Autodesk Fusion 360 part; units mm, degrees
(part 2 of 2)
sketch "lateral-dxf-sketch" plane through (0, 0, 0) normal (0, 1, 0) x (1, 0, 0) in component "Lateral Panel"
  line L0 (153.5, 5) -> (153.5, -5)
  line L1 (153.5, -5) -> (157, -5)
  line L2 (157, -5) -> (157, -15)
  line L3 (157, -15) -> (153.5, -15)
  line L4 (153.5, -15) -> (153.5, -30)
  line L5 (153.5, -30) -> (53.5, -30)
  line L6 (53.5, -30) -> (53.5, 15)
  line L7 (53.5, 15) -> (50, 15)
  line L8 (50, 15) -> (50, -30)
  line L9 (50, -30) -> (-50, -30)
  line L10 (-50, -30) -> (-50, 15)
  line L11 (-50, 15) -> (-53.5, 15)
  line L12 (-53.5, 15) -> (-53.5, -30)
  line L13 (-53.5, -30) -> (-153.5, -30)
  line L14 (-153.5, -30) -> (-153.5, -15)
  line L15 (-153.5, -15) -> (-157, -15)
  line L16 (-157, -15) -> (-157, -5)
  line L17 (-157, -5) -> (-153.5, -5)
  line L18 (-153.5, -5) -> (-153.5, 5)
  line L19 (-153.5, 5) -> (-157, 5)
  line L20 (-157, 5) -> (-157, 15)
  line L21 (-157, 15) -> (-153.5, 15)
  line L22 (-153.5, 15) -> (-153.5, 30)
  line L23 (-153.5, 30) -> (153.5, 30)
  line L24 (153.5, 30) -> (153.5, 15)
  line L25 (153.5, 15) -> (157, 15)
  line L26 (157, 15) -> (157, 5)
  line L27 (157, 5) -> (153.5, 5)
extrude "Extrude1'" add sketch "Sketch1" along normal blind 3.5 separate body makes body 3 in component "Side Panel"
sketch "side-panel-dxf-sketch" plane through (0, 0, 0) normal (0, 1, 0) x (1, 0, 0) in component "Side Panel"
  line L0 (72.2516, -98.9992) -> (68.7516, -98.9992)
  line L1 (68.7516, -98.9992) -> (68.7516, -108.9992)
  line L2 (68.7516, -108.9992) -> (72.2516, -108.9992)
  line L3 (72.2516, -108.9992) -> (72.2516, -98.9992)
  line L4 (213.25, -57) -> (213.25, -47)
  line L5 (213.25, -47) -> (209.75, -47)
  line L6 (209.75, -47) -> (209.75, -57)
  line L7 (209.75, -57) -> (213.25, -57)
  line L8 (213.25, -37) -> (213.25, -27)
  line L9 (213.25, -27) -> (209.75, -27)
  line L10 (209.75, -27) -> (209.75, -37)
  line L11 (209.75, -37) -> (213.25, -37)
  line L12 (189.7503, -38.9999) -> (186.2503, -38.9999)
  line L13 (186.2503, -38.9999) -> (186.2503, -48.9999)
  line L14 (186.2503, -48.9999) -> (189.7503, -48.9999)
  line L15 (189.7503, -48.9999) -> (189.7503, -38.9999)
  line L16 (186.2503, -58.9999) -> (186.2503, -68.9999)
  line L17 (186.2503, -68.9999) -> (189.7503, -68.9999)
  line L18 (189.7503, -68.9999) -> (189.7503, -58.9999)
  line L19 (189.7503, -58.9999) -> (186.2503, -58.9999)
  line L20 (166.2505, -50.9997) -> (162.7505, -50.9997)
  line L21 (162.7505, -50.9997) -> (162.7505, -60.9997)
  line L22 (162.7505, -60.9997) -> (166.2505, -60.9997)
  line L23 (166.2505, -60.9997) -> (166.2505, -50.9997)
  line L24 (162.7505, -70.9997) -> (162.7505, -80.9997)
  line L25 (162.7505, -80.9997) -> (166.2505, -80.9997)
  line L26 (166.2505, -80.9997) -> (166.2505, -70.9997)
  line L27 (166.2505, -70.9997) -> (162.7505, -70.9997)
  line L28 (142.7508, -62.9996) -> (139.2508, -62.9996)
  line L29 (139.2508, -62.9996) -> (139.2508, -72.9996)
  line L30 (139.2508, -72.9996) -> (142.7508, -72.9996)
  line L31 (142.7508, -72.9996) -> (142.7508, -62.9996)
  line L32 (139.2508, -82.9996) -> (139.2508, -92.9996)
  line L33 (139.2508, -92.9996) -> (142.7508, -92.9996)
  line L34 (142.7508, -92.9996) -> (142.7508, -82.9996)
  line L35 (142.7508, -82.9996) -> (139.2508, -82.9996)
  line L36 (119.2511, -74.9995) -> (115.7511, -74.9995)
  line L37 (115.7511, -74.9995) -> (115.7511, -84.9995)
  line L38 (115.7511, -84.9995) -> (119.2511, -84.9995)
  line L39 (119.2511, -84.9995) -> (119.2511, -74.9995)
  line L40 (92.2513, -106.9993) -> (92.2513, -116.9993)
  line L41 (92.2513, -116.9993) -> (95.7513, -116.9993)
  line L42 (95.7513, -116.9993) -> (95.7513, -106.9993)
  line L43 (95.7513, -106.9993) -> (92.2513, -106.9993)
  line L44 (-1.75, -15) -> (-1.75, -25)
  line L45 (-1.75, -25) -> (1.75, -25)
  line L46 (1.75, -25) -> (1.75, -15)
  line L47 (1.75, -15) -> (-1.75, -15)
  line L48 (-1.75, -55) -> (-1.75, -65)
  line L49 (-1.75, -65) -> (1.75, -65)
  line L50 (1.75, -65) -> (1.75, -55)
  line L51 (1.75, -55) -> (-1.75, -55)
  line L52 (95.7513, -86.9993) -> (92.2513, -86.9993)
  line L53 (92.2513, -86.9993) -> (92.2513, -96.9993)
  line L54 (92.2513, -96.9993) -> (95.7513, -96.9993)
  line L55 (95.7513, -96.9993) -> (95.7513, -86.9993)
  line L56 (115.7511, -94.9995) -> (115.7511, -104.9995)
  line L57 (115.7511, -104.9995) -> (119.2511, -104.9995)
  line L58 (119.2511, -104.9995) -> (119.2511, -94.9995)
  line L59 (119.2511, -94.9995) -> (115.7511, -94.9995)
  line L60 (68.7516, -118.9992) -> (68.7516, -128.9992)
  line L61 (68.7516, -128.9992) -> (72.2516, -128.9992)
  line L62 (72.2516, -128.9992) -> (72.2516, -118.9992)
  line L63 (72.2516, -118.9992) -> (68.7516, -118.9992)
  line L64 (45.2519, -130.999) -> (45.2519, -140.999)
  line L65 (45.2519, -140.999) -> (48.7519, -140.999)
  line L66 (48.7519, -140.999) -> (48.7519, -130.999)
  line L67 (48.7519, -130.999) -> (45.2519, -130.999)
  line L68 (25.2521, -122.9989) -> (21.7521, -122.9989)
  line L69 (21.7521, -122.9989) -> (21.7521, -132.9989)
  line L70 (21.7521, -132.9989) -> (25.2521, -132.9989)
  line L71 (25.2521, -132.9989) -> (25.2521, -122.9989)
  line L72 (21.7521, -142.9989) -> (21.7521, -152.9989)
  line L73 (21.7521, -152.9989) -> (25.2521, -152.9989)
  line L74 (25.2521, -152.9989) -> (25.2521, -142.9989)
  line L75 (25.2521, -142.9989) -> (21.7521, -142.9989)
  line L76 (236.75, -45) -> (236.75, -35)
  line L77 (236.75, -35) -> (233.25, -35)
  line L78 (233.25, -35) -> (233.25, -45)
  line L79 (233.25, -45) -> (236.75, -45)
  line L80 (236.75, -5) -> (236.75, 5)
  line L81 (236.75, 5) -> (233.25, 5)
  line L82 (233.25, 5) -> (233.25, -5)
  line L83 (233.25, -5) -> (236.75, -5)
  line L84 (1.75, -145) -> (1.75, -135)
  line L85 (1.75, -135) -> (-1.75, -135)
  line L86 (-1.75, -135) -> (-1.75, -145)
  line L87 (-1.75, -145) -> (1.75, -145)
  line L88 (-1.75, -95) -> (-1.75, -105)
  line L89 (-1.75, -105) -> (1.75, -105)
  line L90 (1.75, -105) -> (1.75, -95)
  line L91 (1.75, -95) -> (-1.75, -95)
  line L92 (48.7519, -110.999) -> (45.2519, -110.999)
  line L93 (45.2519, -110.999) -> (45.2519, -120.999)
  line L94 (45.2519, -120.999) -> (48.7519, -120.999)
  line L95 (48.7519, -120.999) -> (48.7519, -110.999)
  arc A0 (-10, -180) -> (4.5478, -188.9061) centre (0, -180) ccw
  line L96 (-10, -180) -> (-10, 20)
  line L97 (-10, 20) -> (10, 20)
  line L98 (10, 20) -> (10, 12.5)
  arc A1 (10, 12.5) -> (12.5, 10) centre (12.5, 12.5) ccw
  line L99 (12.5, 10) -> (222.4, 10)
  arc A2 (222.4, 10) -> (225, 12.6) centre (222.4, 12.6) ccw
  line L100 (225, 12.6) -> (225, 20)
  line L101 (225, 20) -> (245, 20)
  line L102 (245, 20) -> (245, -60)
  arc A3 (239.5478, -68.9061) -> (245, -60) centre (235, -60) ccw
  line L103 (239.5478, -68.9061) -> (4.5478, -188.9061)
copy_body "CutPasteBodies1" bodies 2 removing the originals makes body 4 in component "Lateral Panel"
extrude "Extrude1''" add sketch "Sketch1 (3)" along normal blind 3.5 separate body makes body 5 in component "Vertical Panels"
sketch "vertical-panel-dxf-sketch" plane through (0, 0, 0) normal (0, 1, 0) x (1, 0, 0) in component "Vertical Panels"
  line L0 (231.5, 143.2128) -> (235, 143.2128)
  line L1 (235, 143.2128) -> (235, 133.2128)
  line L2 (235, 133.2128) -> (231.5, 133.2128)
  line L3 (231.5, 133.2128) -> (231.5, 118.2128)
  line L4 (231.5, 118.2128) -> (0, 0)
  line L5 (0, 0) -> (0, 15)
  line L6 (0, 15) -> (-3.5, 15)
  line L7 (-3.5, 15) -> (-3.5, 25)
  line L8 (-3.5, 25) -> (0, 25)
  line L9 (0, 25) -> (0, 35)
  line L10 (0, 35) -> (-3.5, 35)
  line L11 (-3.5, 35) -> (-3.5, 45)
  line L12 (-3.5, 45) -> (0, 45)
  line L13 (0, 45) -> (0, 60)
  line L14 (0, 60) -> (20.0021, 70.2139)
  line L15 (20.0021, 70.2139) -> (20.0021, 57.0011)
  line L16 (20.0021, 57.0011) -> (23.5021, 57.0011)
  line L17 (23.5021, 57.0011) -> (23.5021, 72.0011)
  line L18 (23.5021, 72.0011) -> (43.5019, 82.2137)
  line L19 (43.5019, 82.2137) -> (43.5019, 69.001)
  line L20 (43.5019, 69.001) -> (47.0019, 69.001)
  line L21 (47.0019, 69.001) -> (47.0019, 84.001)
  line L22 (47.0019, 84.001) -> (67.0016, 94.2136)
  line L23 (67.0016, 94.2136) -> (67.0016, 81.0008)
  line L24 (67.0016, 81.0008) -> (70.5016, 81.0008)
  line L25 (70.5016, 81.0008) -> (70.5016, 96.0008)
  line L26 (70.5016, 96.0008) -> (90.5013, 106.2134)
  line L27 (90.5013, 106.2134) -> (90.5013, 93.0007)
  line L28 (90.5013, 93.0007) -> (94.0013, 93.0007)
  line L29 (94.0013, 93.0007) -> (94.0013, 108.0007)
  line L30 (94.0013, 108.0007) -> (114.0011, 118.2133)
  line L31 (114.0011, 118.2133) -> (114.0011, 105.0005)
  line L32 (114.0011, 105.0005) -> (117.5011, 105.0005)
  line L33 (117.5011, 105.0005) -> (117.5011, 120.0005)
  line L34 (117.5011, 120.0005) -> (137.5008, 130.2132)
  line L35 (137.5008, 130.2132) -> (137.5008, 117.0004)
  line L36 (137.5008, 117.0004) -> (141.0008, 117.0004)
  line L37 (141.0008, 117.0004) -> (141.0008, 132.0004)
  line L38 (141.0008, 132.0004) -> (161.0005, 142.213)
  line L39 (161.0005, 142.213) -> (161.0005, 129.0003)
  line L40 (161.0005, 129.0003) -> (164.5005, 129.0003)
  line L41 (164.5005, 129.0003) -> (164.5005, 144.0003)
  line L42 (164.5005, 144.0003) -> (184.5003, 154.2129)
  line L43 (184.5003, 154.2129) -> (184.5003, 141.0001)
  line L44 (184.5003, 141.0001) -> (188.0003, 141.0001)
  line L45 (188.0003, 141.0001) -> (188.0003, 156.0001)
  line L46 (188.0003, 156.0001) -> (208, 166.2128)
  line L47 (208, 166.2128) -> (208, 153)
  line L48 (208, 153) -> (211.5, 153)
  line L49 (211.5, 153) -> (211.5, 168)
  line L50 (211.5, 168) -> (231.5, 178.2128)
  line L51 (231.5, 178.2128) -> (231.5, 163.2128)
  line L52 (231.5, 163.2128) -> (235, 163.2128)
  line L53 (235, 163.2128) -> (235, 153.2128)
  line L54 (235, 153.2128) -> (231.5, 153.2128)
  line L55 (231.5, 153.2128) -> (231.5, 143.2128)
extrude "Extrude1'''" add sketch "Sketch1 (4)" along normal blind 3.5 separate body makes body 6 in component "Front Panels"
sketch "front-panel-dxf-sketch" plane through (0, 0, 0) normal (0, 1, 0) x (1, 0, 0) in component "Front Panels"
  line L0 (-53.5, -20) -> (-53.5, -30)
  line L1 (-53.5, -30) -> (-50, -30)
  line L2 (-50, -30) -> (-50, -20)
  line L3 (-50, -20) -> (-53.5, -20)
  line L4 (-50, 0) -> (-53.5, 0)
  line L5 (-53.5, 0) -> (-53.5, -10)
  line L6 (-53.5, -10) -> (-50, -10)
  line L7 (-50, -10) -> (-50, 0)
  line L8 (53.5, 0) -> (50, 0)
  line L9 (50, 0) -> (50, -10)
  line L10 (50, -10) -> (53.5, -10)
  line L11 (53.5, -10) -> (53.5, 0)
  line L12 (68.5, 16.6542) -> (88.5, 16.6542)
  line L13 (88.5, 16.6542) -> (88.5, 23.3458)
  line L14 (88.5, 23.3458) -> (68.5, 23.3458)
  line L15 (68.5, 23.3458) -> (68.5, 16.6542)
  line L16 (31, 23.3458) -> (31, 16.6542)
  line L17 (31, 16.6542) -> (51, 16.6542)
  line L18 (51, 16.6542) -> (51, 23.3458)
  line L19 (51, 23.3458) -> (31, 23.3458)
  line L20 (-51, 23.3458) -> (-51, 16.6542)
  line L21 (-51, 16.6542) -> (-31, 16.6542)
  line L22 (-31, 16.6542) -> (-31, 23.3458)
  line L23 (-31, 23.3458) -> (-51, 23.3458)
  line L24 (53.5, -20) -> (50, -20)
  line L25 (50, -20) -> (50, -30)
  line L26 (50, -30) -> (53.5, -30)
  line L27 (53.5, -30) -> (53.5, -20)
  line L28 (106, 16.6542) -> (126, 16.6542)
  line L29 (126, 16.6542) -> (126, 23.3458)
  line L30 (126, 23.3458) -> (106, 23.3458)
  line L31 (106, 23.3458) -> (106, 16.6542)
  line L32 (-88.5, 23.3458) -> (-88.5, 16.6542)
  line L33 (-88.5, 16.6542) -> (-68.5, 16.6542)
  line L34 (-68.5, 16.6542) -> (-68.5, 23.3458)
  line L35 (-68.5, 23.3458) -> (-88.5, 23.3458)
  line L36 (-106, 16.6542) -> (-106, 23.3458)
  line L37 (-106, 23.3458) -> (-126, 23.3458)
  line L38 (-126, 23.3458) -> (-126, 16.6542)
  line L39 (-126, 16.6542) -> (-106, 16.6542)
  line L40 (153.5, -25) -> (153.5, -40)
  line L41 (153.5, -40) -> (-153.5, -40)
  line L42 (-153.5, -40) -> (-153.5, -25)
  line L43 (-153.5, -25) -> (-157, -25)
  line L44 (-157, -25) -> (-157, -15)
  line L45 (-157, -15) -> (-153.5, -15)
  line L46 (-153.5, -15) -> (-153.5, 15)
  line L47 (-153.5, 15) -> (-157, 15)
  line L48 (-157, 15) -> (-157, 25)
  line L49 (-157, 25) -> (-153.5, 25)
  line L50 (-153.5, 25) -> (-153.5, 40)
  line L51 (-153.5, 40) -> (153.5, 40)
  line L52 (153.5, 40) -> (153.5, 25)
  line L53 (153.5, 25) -> (157, 25)
  line L54 (157, 25) -> (157, 15)
  line L55 (157, 15) -> (153.5, 15)
  line L56 (153.5, 15) -> (153.5, -15)
  line L57 (153.5, -15) -> (157, -15)
  line L58 (157, -15) -> (157, -25)
  line L59 (157, -25) -> (153.5, -25)
extrude "Extrude1''''" add sketch "Sketch2" along normal blind 3.5 separate body contours L0 L2 L7 L8 L9 L10 L11 L13 L14 L15 L17 L18 L19 L21 L23 L26 L27 L28 L29 L31 L32 L34 L35 L36 L37 L38 L52 L53 L54 L55 L56 L57 L58 L59 L60 L61 L111 | L94 L95 L96 L97 | L99 L100 L101 L102 | L103 L107 L108 L109 | L104 L105 L106 L110 makes body 7 in component "Back Panel"
extrude "Extrude1'''''" add sketch "Sketch1 (6)" along normal blind 3.5 separate body makes body 8 in component "Bottom Panel"
sketch "bottom-dxf-sketch" plane through (0, 0, 0) normal (0, 1, 0) x (1, 0, 0) in component "Bottom Panel"
  line L0 (-31, 131.4299) -> (-31, 127.5)
  line L1 (-31, 127.5) -> (31, 127.5)
  line L2 (31, 127.5) -> (31, 131.4299)
  line L3 (31, 131.4299) -> (51, 131.4299)
  line L4 (51, 131.4299) -> (51, 127.5)
  line L5 (51, 127.5) -> (68.5, 127.5)
  line L6 (68.5, 127.5) -> (68.5, 131.4299)
  line L7 (68.5, 131.4299) -> (88.5, 131.4299)
  line L8 (88.5, 131.4299) -> (88.5, 127.5)
  line L9 (88.5, 127.5) -> (106, 127.5)
  line L10 (106, 127.5) -> (106, 131.4299)
  line L11 (106, 131.4299) -> (126, 131.4299)
  line L12 (126, 131.4299) -> (126, 127.5)
  line L13 (126, 127.5) -> (153.5, 127.5)
  line L14 (153.5, 127.5) -> (153.5, -127.5)
  line L15 (153.5, -127.5) -> (126, -127.5)
  line L16 (126, -127.5) -> (126, -131.4299)
  line L17 (126, -131.4299) -> (106, -131.4299)
  line L18 (106, -131.4299) -> (106, -127.5)
  line L19 (106, -127.5) -> (88.5, -127.5)
  line L20 (88.5, -127.5) -> (88.5, -131.4299)
  line L21 (88.5, -131.4299) -> (68.5, -131.4299)
  line L22 (68.5, -131.4299) -> (68.5, -127.5)
  line L23 (68.5, -127.5) -> (51, -127.5)
  line L24 (51, -127.5) -> (51, -131.4299)
  line L25 (51, -131.4299) -> (31, -131.4299)
  line L26 (31, -131.4299) -> (31, -127.5)
  line L27 (31, -127.5) -> (-31, -127.5)
  line L28 (-31, -127.5) -> (-31, -131.4299)
  line L29 (-31, -131.4299) -> (-51, -131.4299)
  line L30 (-51, -131.4299) -> (-51, -127.5)
  line L31 (-51, -127.5) -> (-68.5, -127.5)
  line L32 (-68.5, -127.5) -> (-68.5, -131.4299)
  line L33 (-68.5, -131.4299) -> (-88.5, -131.4299)
  line L34 (-88.5, -131.4299) -> (-88.5, -127.5)
  line L35 (-88.5, -127.5) -> (-106, -127.5)
  line L36 (-106, -127.5) -> (-106, -131.4299)
  line L37 (-106, -131.4299) -> (-126, -131.4299)
  line L38 (-126, -131.4299) -> (-126, -127.5)
  line L39 (-126, -127.5) -> (-153.5, -127.5)
  line L40 (-153.5, -127.5) -> (-153.5, 127.5)
  line L41 (-153.5, 127.5) -> (-126, 127.5)
  line L42 (-126, 127.5) -> (-126, 131.4299)
  line L43 (-126, 131.4299) -> (-106, 131.4299)
  line L44 (-106, 131.4299) -> (-106, 127.5)
  line L45 (-106, 127.5) -> (-88.5, 127.5)
  line L46 (-88.5, 127.5) -> (-88.5, 131.4299)
  line L47 (-88.5, 131.4299) -> (-68.5, 131.4299)
  line L48 (-68.5, 131.4299) -> (-68.5, 127.5)
  line L49 (-68.5, 127.5) -> (-51, 127.5)
  line L50 (-51, 127.5) -> (-51, 131.4299)
  line L51 (-51, 131.4299) -> (-31, 131.4299)
extrude "Extrude3" add sketch "Sketch2" along normal blind 3.5 contours L2 L111 L112 L113 L114 bodies 1 7 in component "Back Panel"
extrude "Extrude4" cut sketch "Sketch2" along normal up to surface (3.5 mm away) contours L94 L95 L96 L97 | L99 L100 L101 L102 | L103 L107 L108 L109 | L104 L105 L106 L110 bodies 1 in component "Back Panel"
sketch "back-panel-dxf-sketch" plane through (0, 0, 0) normal (0, 1, 0) x (1, 0, 0) in component "Back Panel"
  line L0 (50, -60) -> (50, -70)
  line L1 (50, -70) -> (53.5, -70)
  line L2 (53.5, -70) -> (53.5, -60)
  line L3 (53.5, -60) -> (50, -60)
  line L4 (-53.5, -70) -> (-50, -70)
  line L5 (-50, -70) -> (-50, -60)
  line L6 (-50, -60) -> (-53.5, -60)
  line L7 (-53.5, -60) -> (-53.5, -70)
  line L8 (50, -80) -> (50, -90)
  line L9 (50, -90) -> (53.5, -90)
  line L10 (53.5, -90) -> (53.5, -80)
  line L11 (53.5, -80) -> (50, -80)
  line L12 (-53.5, -90) -> (-50, -90)
  line L13 (-50, -90) -> (-50, -80)
  line L14 (-50, -80) -> (-53.5, -80)
  line L15 (-53.5, -80) -> (-53.5, -90)
  line L16 (88.5, -36.6542) -> (68.5, -36.6542)
  line L17 (68.5, -36.6542) -> (68.5, -43.3458)
  line L18 (68.5, -43.3458) -> (88.5, -43.3458)
  line L19 (88.5, -43.3458) -> (88.5, -36.6542)
  line L20 (106, -43.3458) -> (126, -43.3458)
  line L21 (126, -43.3458) -> (126, -36.6542)
  line L22 (126, -36.6542) -> (106, -36.6542)
  line L23 (106, -36.6542) -> (106, -43.3458)
  line L24 (31, -43.3458) -> (51, -43.3458)
  line L25 (51, -43.3458) -> (51, -36.6542)
  line L26 (51, -36.6542) -> (31, -36.6542)
  line L27 (31, -36.6542) -> (31, -43.3458)
  line L28 (-106, -43.3458) -> (-106, -36.6542)
  line L29 (-106, -36.6542) -> (-126, -36.6542)
  line L30 (-126, -36.6542) -> (-126, -43.3458)
  line L31 (-126, -43.3458) -> (-106, -43.3458)
  line L32 (-51, -43.3458) -> (-31, -43.3458)
  line L33 (-31, -43.3458) -> (-31, -36.6542)
  line L34 (-31, -36.6542) -> (-51, -36.6542)
  line L35 (-51, -36.6542) -> (-51, -43.3458)
  line L36 (-88.5, -43.3458) -> (-68.5, -43.3458)
  line L37 (-68.5, -43.3458) -> (-68.5, -36.6542)
  line L38 (-68.5, -36.6542) -> (-88.5, -36.6542)
  line L39 (-88.5, -36.6542) -> (-88.5, -43.3458)
  line L40 (153.5, -65) -> (153.5, -105)
  line L41 (153.5, -105) -> (-153.5, -105)
  line L42 (-153.5, -105) -> (-153.5, -65)
  line L43 (-153.5, -65) -> (-157, -65)
  line L44 (-157, -65) -> (-157, -55)
  line L45 (-157, -55) -> (-153.5, -55)
  line L46 (-153.5, -55) -> (-153.5, -25)
  line L47 (-153.5, -25) -> (-157, -25)
  line L48 (-157, -25) -> (-157, -15)
  line L49 (-157, -15) -> (-153.5, -15)
  line L50 (-153.5, -15) -> (-153.5, 15)
  line L51 (-153.5, 15) -> (-157, 15)
  line L52 (-157, 15) -> (-157, 25)
  line L53 (-157, 25) -> (-153.5, 25)
  line L54 (-153.5, 25) -> (-153.5, 55)
  line L55 (-153.5, 55) -> (-157, 55)
  line L56 (-157, 55) -> (-157, 65)
  line L57 (-157, 65) -> (-153.5, 65)
  line L58 (-153.5, 65) -> (-153.5, 100)
  line L59 (-153.5, 100) -> (153.5, 100)
  line L60 (153.5, 100) -> (153.5, 65)
  line L61 (153.5, 65) -> (157, 65)
  line L62 (157, 65) -> (157, 55)
  line L63 (157, 55) -> (153.5, 55)
  line L64 (153.5, 55) -> (153.5, 25)
  line L65 (153.5, 25) -> (157, 25)
  line L66 (157, 25) -> (157, 15)
  line L67 (157, 15) -> (153.5, 15)
  line L68 (153.5, 15) -> (153.5, -15)
  line L69 (153.5, -15) -> (157, -15)
  line L70 (157, -15) -> (157, -25)
  line L71 (157, -25) -> (153.5, -25)
  line L72 (153.5, -25) -> (153.5, -55)
  line L73 (153.5, -55) -> (157, -55)
  line L74 (157, -55) -> (157, -65)
  line L75 (157, -65) -> (153.5, -65)
component "Lateral Panel" placed x (1, 0, 0) y (0, 1, 0) z (0, 0, 1) at (0, 0, 0)
component "Side Panel" placed x (1, 0, 0) y (0, 1, 0) z (0, 0, 1) at (0, 0, 0)
component "Vertical Panels" placed x (1, 0, 0) y (0, 1, 0) z (0, 0, 1) at (0, 0, 0)
component "Front Panels" placed x (1, 0, 0) y (0, 1, 0) z (0, 0, 1) at (0, 0, 0)
component "Back Panel" placed x (1, 0, 0) y (0, 1, 0) z (0, 0, 1) at (0, 0, 0)
component "Bottom Panel" placed x (1, 0, 0) y (0, 1, 0) z (0, 0, 1) at (0, 0, 0)
equation "d44 = inclination_angle"
equation "d45 = 23.5 cm - 0.35 cm"
equation "d65 = 6 cm - 4.5 cm"
equation "d117 = ( 2 * 0.35 * tan(inclination_angle) ) * 1 cm + ( 0.35 * cos(inclination_angle) ) * 1 cm"
equation "inclination_angle = atan(12 / 23.5)"
equation "d132 = ( 2 * 0.35 * tan(inclination_angle) ) * 1 cm + ( 0.35 * cos(inclination_angle) ) * 1 cm"
equation "d140 = ( 0.35 / cos(inclination_angle) ) * 1 cm"
